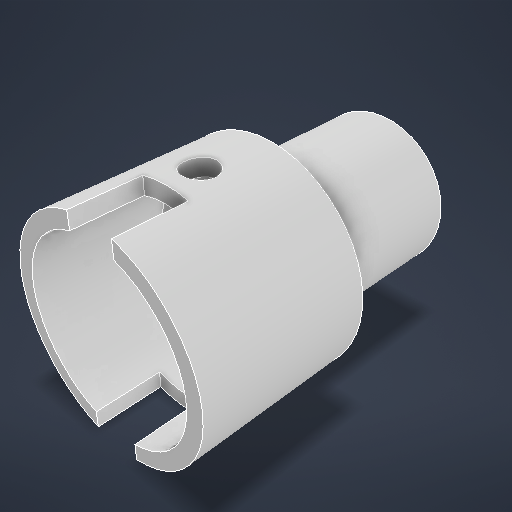
# Autodesk Inventor part: Wheel_Lego_Axle_Connector
Saved by Autodesk Inventor 2025 (Build 290162000, 162)
## iProperties
Created: 2024-06-03
Part Number: Wheel_Lego_Axle_Connector
Material: Generic
Document SubType Name: Modeling
Designer: Garfieldcmix
Density: 1 g/cm^3
Appearance: Default
Author: Garfieldcmix
Autodesk Inventor part; units mm, degrees
ref_plane "YZ Plane" through (0, 0, 0) normal (1, 0, 0) x (0, 1, 0)
ref_plane "XY Plane" through (0, 0, 0) normal (0, 0, 1) x (1, 0, 0)
derived "Motor_Lego_Axle_Connector.ipt"
sketch "Motor_Lego_Axle_Connector" plane through (0, 0, 0) normal (0, 0, 1) x (1, 0, 0)
  circle A0 centre (0, 0) radius 4.5
  circle A1 centre (0, 0) radius 2.7
  line L0 (-1.8, 2.0125) -> (-1.8, -2.0125)
  line L1 (0, 4.5) -> (0, -4.5) construction
  line L2 (1.8, 2.0125) -> (1.8, -2.0125)
  line L3 (0.9, 2.4) -> (-0.9, 2.4)
  line L4 (0.9, 2.4) -> (0.9, 1.4)
  line L5 (1.4, 1.4) -> (0.9, 1.4) construction
  line L6 (1.4, 1.4) -> (1.4, 0.9) construction
  arc A2 (0.9, 1.4) -> (1.4, 0.9) centre (1.4, 1.4) ccw
  line L7 (1.4, 0.9) -> (2.4, 0.9)
  line L8 (-0.9, 1.4) -> (-0.9, 2.4)
  arc A3 (-1.4, 0.9) -> (-0.9, 1.4) centre (-1.4, 1.4) ccw
  line L9 (-2.4, 0.9) -> (-1.4, 0.9)
  line L10 (-2.4, 0.9) -> (-2.4, -0.9)
  line L11 (-1.4, -0.9) -> (-2.4, -0.9)
  arc A4 (-0.9, -1.4) -> (-1.4, -0.9) centre (-1.4, -1.4) ccw
  line L12 (-0.9, -2.4) -> (-0.9, -1.4)
  line L13 (-0.9, -2.4) -> (0.9, -2.4)
  line L14 (0.9, -1.4) -> (0.9, -2.4)
  arc A5 (1.4, -0.9) -> (0.9, -1.4) centre (1.4, -1.4) ccw
  line L15 (2.4, -0.9) -> (1.4, -0.9)
  line L16 (2.4, -0.9) -> (2.4, 0.9)
  point P0 (0, 2.4)
  point P1 (-2.4, 0)
  point P2 (0, -2.4)
  point P3 (2.4, 0)
sketch "Wheel_Lego_Axle_Connector" plane through (0, 0, 0) normal (0, 0, 1) x (1, 0, 0)
  circle A0 centre (0, 0) radius 4.5 projected
  circle A1 centre (0, 0) radius 2.7 projected
  line L0 (-0.9, 1.4) -> (-0.9, 2.4) projected
  line L1 (0.9, 2.4) -> (-0.9, 2.4) projected
  line L2 (0.9, 2.4) -> (0.9, 1.4) projected
  arc A2 (0.9, 1.4) -> (1.4, 0.9) centre (1.4, 1.4) ccw projected
  line L3 (1.4, 0.9) -> (2.4, 0.9) projected
  line L4 (2.4, -0.9) -> (2.4, 0.9) projected
  line L5 (2.4, -0.9) -> (1.4, -0.9) projected
  arc A3 (1.4, -0.9) -> (0.9, -1.4) centre (1.4, -1.4) ccw projected
  line L6 (0.9, -1.4) -> (0.9, -2.4) projected
  line L7 (-0.9, -2.4) -> (0.9, -2.4) projected
  line L8 (-0.9, -2.4) -> (-0.9, -1.4) projected
  arc A4 (-0.9, -1.4) -> (-1.4, -0.9) centre (-1.4, -1.4) ccw projected
  line L9 (-1.4, -0.9) -> (-2.4, -0.9) projected
  line L10 (-2.4, 0.9) -> (-2.4, -0.9) projected
  line L11 (-2.4, 0.9) -> (-1.4, 0.9) projected
  arc A5 (-1.4, 0.9) -> (-0.9, 1.4) centre (-1.4, 1.4) ccw projected
  circle A6 centre (0, 0) radius 6.5
  circle A7 centre (0, 0) radius 5.5
  dimension "d1" = 13
  dimension "d10" = 11
  constraints: 2 centre point, 2 coincident
  measures "d1" diameter of A6
  measures "d10" diameter of A7
extrude "Seperator_Extrusion" add sketch "Wheel_Lego_Axle_Connector" against normal blind 2 contours A0 | A1 | L0 L1 L2 A2 L3 L4 L5 A3 L6 L7 L8 A4 L9 L10 L11 A5 | A6 | A7
extrude "Lego_Axle_Connector_Extrusion" add sketch "Wheel_Lego_Axle_Connector" against normal blind 11 contours A0 | A1
extrude "Extrusion4" add sketch "Wheel_Lego_Axle_Connector" along normal blind 8 contours A6
ref_plane "Work Plane1" through (0, 6.5, 0) normal (0, 1, 0) x (-1, 0, 0)
sketch "Sketch3" plane through (0, 6.5, 0) normal (0, 1, 0) x (-1, 0, 0)
  circle A0 centre (0, 2) radius 1
  line L0 (6.5, 8) -> (-6.5, 8) construction
  line L1 (0, 8) -> (0, 0) construction
  line L2 (1.5, 8) -> (1.5, 4)
  line L3 (1.5, 4) -> (-1.5, 4)
  line L4 (-1.5, 4) -> (-1.5, 8)
  line L5 (1.5, 8) -> (-1.5, 8)
  point P0 (0, 4)
  dimension "d13" = 2
  dimension "d17" = 6
  dimension "d18" = 3
  dimension "d19" = 4
  constraints: 10 end point, 3 midpoint, 3 perpendicular, 3 point on line, 1 centre point, 1 collinear, 1 vertical
  measures "d13" diameter of A0
  measures "d17" distance from line of A0.centre L0
  measures "d18" distance between parallel lines of L4 L2
  measures "d19" distance from line of L0 point (0, 4)
extrude "Extrusion5" cut sketch "Sketch3" against normal through all
sketch "Connector_Sketch" plane through (0, 0, 8) normal (0, 0, 1) x (1, 0, 0)
  line L0 (-1.5, -6.3246) -> (-1.5, -5.2915) projected
  arc A0 (-1.5, 5.2915) -> (-1.5, -5.2915) centre (0, 0) ccw projected
  line L1 (-1.5, 5.2915) -> (-1.5, 6.3246) projected
  arc A1 (-1.5, 6.3246) -> (-1.5, -6.3246) centre (0, 0) ccw projected
  line L2 (1.5, -5.2915) -> (1.5, -6.3246) projected
  arc A2 (1.5, -6.3246) -> (1.5, 6.3246) centre (0, 0) ccw projected
  line L3 (1.5, 6.3246) -> (1.5, 5.2915) projected
  arc A3 (1.5, -5.2915) -> (1.5, 5.2915) centre (0, 0) ccw projected
sketch "Connector_2_Sketch" plane through (0, 6.5, 0) normal (0, 1, 0) x (-1, 0, 0)
  line L0 (-1.5, 4) -> (1.5, 4) projected
  line L1 (1.5, 8) -> (1.5, 4) projected
  line L2 (-1.5, 4) -> (-1.5, 8) projected
  line L3 (1.5, 8) -> (-1.5, 8)
  constraints: 2 end point, 2 vertical alignment, 1 horizontal
ref_plane "Work Plane2" through (0, -6.5, 0) normal (0, 1, 0) x (-1, 0, 0)
sketch "Connector_3_Sketch" plane through (0, -6.5, 0) normal (0, 1, 0) x (-1, 0, 0)
  line L0 (1.5, 8) -> (1.5, 4) projected
  line L1 (-1.5, 4) -> (1.5, 4) projected
  line L2 (-1.5, 8) -> (-1.5, 4) projected
  line L3 (1.5, 8) -> (1.5, 4) projected
  line L4 (1.5, 8) -> (-1.5, 8)
  constraints: 2 end point, 1 perpendicular
body "Solid1"
